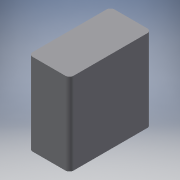
# Autodesk Inventor part: USB_Cap
Saved by Autodesk Inventor 2016 (Build 200138000, 138)
## iProperties
Created: 2017-07-18
Part Number: USB_Cap
Material: Generic
Document SubType Name: Modeling
Designer: bobbyl
Density: 1 g/cm^3
Appearance: Default
Author: bobbyl
Autodesk Inventor part; units mm, degrees
ref_plane "YZ Plane" through (0, 0, 0) normal (1, 0, 0) x (0, 1, 0)
ref_plane "XZ Plane" through (0, 0, 0) normal (0, 1, 0) x (-1, 0, 0)
ref_plane "XY Plane" through (0, 0, 0) normal (0, 0, 1) x (1, 0, 0)
sketch "Sketch1" plane through (0, 0, 0) normal (0, 0, 1) x (1, 0, 0)
  line L0 (11.25, -5) -> (1.25, -5) projected
  line L1 (1.25, -5) -> (1.25, 30) projected
  line L2 (1.25, 30) -> (11.25, 30) projected
  line L3 (11.25, 30) -> (11.25, -5) projected
  arc A0 (16.25, -12.5) -> (18.75, -10) centre (16.25, -10) ccw projected
  line L4 (18.75, -10) -> (18.75, 35) projected
  arc A1 (18.75, 35) -> (16.25, 37.5) centre (16.25, 35) ccw projected
  line L5 (16.25, 37.5) -> (-3.75, 37.5) projected
  arc A2 (-3.75, 37.5) -> (-6.25, 35) centre (-3.75, 35) ccw projected
  line L6 (-6.25, 35) -> (-6.25, -10) projected
  arc A3 (-6.25, -10) -> (-3.75, -12.5) centre (-3.75, -10) ccw projected
  line L7 (-3.75, -12.5) -> (16.25, -12.5) projected
  line L8 (-6.25, -10) -> (-6.25, 35)
  arc A4 (-3.75, 37.5) -> (-6.25, 35) centre (-3.75, 35) ccw
  line L9 (-3.75, 37.5) -> (16.25, 37.5)
  arc A5 (18.75, 35) -> (16.25, 37.5) centre (16.25, 35) ccw
  line L10 (18.75, 35) -> (18.75, -10)
  arc A6 (16.25, -12.5) -> (18.75, -10) centre (16.25, -10) ccw
  line L11 (16.25, -12.5) -> (-3.75, -12.5)
  arc A7 (-6.25, -10) -> (-3.75, -12.5) centre (-3.75, -10) ccw
  point P0 (0, 0)
  dimension "d0" = 0
  constraints: 8 end point, 8 point on circle, 4 centre point, 7 other
  measures "d0" distance between parallel lines of L6 L8
extrude "Extrusion1" add sketch "Sketch1" along normal blind 40 contours L0 L1 L2 L3 | L7 A3 L6 A2 L5 A1 L4 A0
sketch "Sketch2" plane through (0, 0, 0) normal (0, 0, -1) x (-1, 0, 0)
  line L0 (-16.25, -10) -> (-16.25, 35) projected
  line L1 (3.75, -10) -> (-16.25, -10) projected
  line L2 (3.75, 35) -> (3.75, -10) projected
  line L3 (-16.25, 35) -> (3.75, 35) projected
  line L4 (-11.25, -5) -> (-11.25, 30) projected
  line L5 (-11.25, 30) -> (-1.25, 30) projected
  line L6 (-1.25, 30) -> (-1.25, -5) projected
  line L7 (-1.25, -5) -> (-11.25, -5) projected
  line L8 (-2.75, 28.5) -> (-9.75, 28.5) projected
  line L9 (-9.75, 28.5) -> (-9.75, -3.5) projected
  line L10 (-9.75, -3.5) -> (-2.75, -3.5) projected
  line L11 (-2.75, -3.5) -> (-2.75, 28.5) projected
  line L12 (-1.25, -5) -> (-11.25, -5)
  line L13 (-11.25, -5) -> (-11.25, 30)
  line L14 (-11.25, 30) -> (-1.25, 30)
  line L15 (-1.25, 30) -> (-1.25, -5)
  point P0 (0, 0)
  constraints: 8 end point, 2 parallel, 1 horizontal, 1 perpendicular
extrude "Extrusion2" cut sketch "Sketch2" against normal blind 30 contours L4 L5 L6 L7 | L11 L10 L9 L8
body "Solid1"
